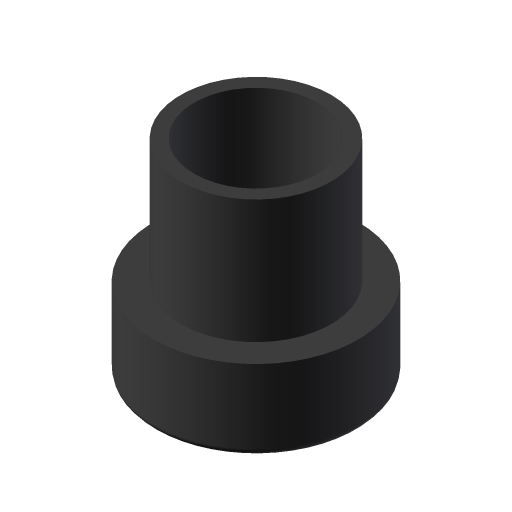
# Autodesk Inventor part: scoringelement
Saved by Autodesk Inventor 2023 (Build 270158000, 158)
## iProperties
Created: 2022-11-04
Part Number: scoringelement
Material: Generic
Document SubType Name: Modeling
Designer: myan
Density: 1 g/cm^3
Appearance: Default
Author: myan
Autodesk Inventor part; units mm, degrees
ref_plane "YZ Plane" through (0, 0, 0) normal (1, 0, 0) x (0, 1, 0)
ref_plane "XZ Plane" through (0, 0, 0) normal (0, 1, 0) x (-1, 0, 0)
ref_plane "XY Plane" through (0, 0, 0) normal (0, 0, 1) x (1, 0, 0)
sketch "Sketch3" plane through (0, 0, 0) normal (1, 0, 0) x (0, 1, 0)
  line L0 (106.9822, -49.7666) -> (49.1134, -49.7666)
  line L1 (48.5622, -49.7666) -> (48.5622, -56.1166)
  line L2 (48.5622, -56.1166) -> (106.9822, -56.1166)
  line L3 (106.9822, -56.1166) -> (106.9822, -49.7666)
  line L4 (117.2485, -20.5566) -> (31.2073, -20.5566)
  line L5 (48.5622, -49.7666) -> (48.5622, -68.8166)
  line L6 (48.5622, -68.8166) -> (13.6372, -68.8166)
  line L7 (12.5671, -62.6523) -> (48.0433, -49.9523)
  arc A0 (12.5671, -62.6523) -> (13.6372, -68.8166) centre (13.6372, -65.6416) ccw
  arc A1 (49.1134, -49.7666) -> (48.0433, -49.9523) centre (49.1134, -52.9416) ccw
  point P0 (0, 0)
  point P1 (48.5622, -56.1166)
  point P2 (64.2516, -56.2504)
  point P3 (48.5622, -49.8148)
  dimension "d13" = 58.42
  dimension "d14" = 6.35
  dimension "d15" = 12.7
  dimension "d17" = 48.26
  dimension "d35" = 3.175
  dimension "d36" = 38.1
  dimension "d37" = 3.175
  constraints: 16 end point, 4 point on circle, 4 tangent, 2 centre point, 2 horizontal, 2 parallel, 2 perpendicular, 2 point on line, 1 vertical
  measures "d13" distance of L1.end L2.end
  measures "d14" distance of L1.start L1.end
  measures "d15" distance between parallel lines of L2 L6
  measures "d17" distance between parallel lines of L4 L6
  measures "d35" radius of A0
  measures "d37" radius of A1
revolve "Revolution2" add sketch "Sketch3" angle 360 about axis through (0, 117.2485, -20.5566) along (0, -1, 0)
body "Solid2"
